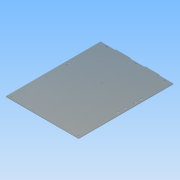
# Autodesk Inventor part: задняя  панель new
Saved by Autodesk Inventor 2017 (Build 210142000, 142)
## iProperties
Part Number: задняя  панель new
Material: Типовые
Document SubType Name: Modeling
Designer: Max
Mass: 792.41 g
Surface Area: 4047.62 cm^2
Volume: 792.41 cm^3
Density: 1 g/cm^3
Appearance: Поликарбонат — дымчатый
Author: Max
Autodesk Inventor part; units mm, degrees
ref_plane "YZ Plane" through (0, 0, 0) normal (1, 0, 0) x (0, 1, 0)
ref_plane "XZ Plane" through (0, 0, 0) normal (0, 1, 0) x (-1, 0, 0)
ref_plane "XY Plane" through (0, 0, 0) normal (0, 0, 1) x (1, 0, 0)
sketch "Эскиз1" plane through (0, 0, 0) normal (0, 0, 1) x (1, 0, 0)
  circle A0 centre (7.4641, 67.6713) radius 2
  circle A1 centre (7.4641, 364.6713) radius 2
  circle A2 centre (-351.5359, 364.6713) radius 2
  circle A3 centre (-351.5359, 67.6713) radius 2
  line L0 (-359.0359, 370.6713) -> (14.9641, 370.6713)
  line L1 (14.9641, 370.6713) -> (14.9641, 53.6713)
  line L2 (14.9641, 53.6713) -> (-359.0359, 53.6713)
  line L3 (-359.0359, 53.6713) -> (-359.0359, 370.6713)
  line L4 (-359.0359, 370.6713) -> (-367.0359, 370.6713)
  line L5 (-367.0359, 370.6713) -> (-367.0359, 53.6713)
  line L6 (-367.0359, 53.6713) -> (-359.0359, 53.6713)
  line L7 (-359.0359, 53.6713) -> (-359.0359, 370.6713)
  line L8 (14.9641, 370.6713) -> (22.9641, 370.6713)
  line L9 (22.9641, 370.6713) -> (22.9641, 53.6713)
  line L10 (22.9641, 53.6713) -> (14.9641, 53.6713)
  line L11 (14.9641, 53.6713) -> (14.9641, 370.6713)
  dimension "d4" = 374
  dimension "d6" = 317
  dimension "d7" = 14
  dimension "d40" = 7.5
  dimension "d41" = 297
  dimension "d42" = 7.5
  dimension "d43" = 7.5
  dimension "d44" = 297
  dimension "d45" = 6
  dimension "d46" = 359
  dimension "d47" = 14
  dimension "d48" = 359
  dimension "d66" = 8
  dimension "d67" = 8
  dimension "d68" = 390
  dimension "d92" = 4
  dimension "d93" = 4
  dimension "d94" = 4
  dimension "d95" = 4
  constraints: 24 end point, 6 parallel, 4 centre point, 3 horizontal, 3 perpendicular, 1 coincident, 1 point on line
  measures "d4" distance between parallel lines of L1 L3
  measures "d6" distance between parallel lines of L0 L2
  measures "d7" distance from line of A3.centre L2
  measures "d40" distance from line of L1 A0.centre
  measures "d41" distance of A0.centre A1.centre
  measures "d42" distance from line of L1 A1.centre
  measures "d43" distance from line of L3 A2.centre
  measures "d44" distance of A3.centre A2.centre
  measures "d45" distance from line of L0 A2.centre
  measures "d46" distance of A0.centre A3.centre
  measures "d47" distance from line of L2 A0.centre
  measures "d48" distance of A1.centre A2.centre
  measures "d66" distance between parallel lines of L9 L1
  measures "d67" distance between parallel lines of L7 L5
  measures "d68" distance between parallel lines of L5 L9
  measures "d92" diameter of A3
  measures "d93" diameter of A0
  measures "d94" diameter of A1
  measures "d95" diameter of A2
extrude "Выдавливание1" add sketch "Эскиз1" along normal blind 4
sketch "Эскиз3" plane through (0, 0, 4) normal (0, 0, 1) x (1, 0, 0)
  circle A0 centre (7.4641, 319.6713) radius 5
  circle A1 centre (7.4641, 282.6713) radius 5
  circle A2 centre (-351.5359, 254.6713) radius 2
  point P0 (0, 0)
  dimension "d96" = 10
  dimension "d97" = 10
  constraints: 3 centre point, 4 other
  measures "d96" diameter of A0
  measures "d97" diameter of A1
sketch "Эскиз4" plane through (0, 0, 4) normal (0, 0, 1) x (1, 0, 0)
  circle A0 centre (-171.5359, 372.6713) radius 1.5
  line L0 (-182.5359, 370.6713) -> (-179.0359, 378.6713)
  line L1 (-179.0359, 378.6713) -> (-164.0359, 378.6713)
  line L2 (-164.0359, 378.6713) -> (-160.5359, 370.6713)
  line L3 (22.9641, 370.6713) -> (-367.0359, 370.6713) projected
  line L4 (-171.5359, 372.6713) -> (-171.5359, 378.6713)
  circle A1 centre (-171.5359, 372.6713) radius 1.5
  point P0 (0, 0)
  point P1 (10.9641, 370.6713)
  point P2 (-363.0359, 370.6713)
  dimension "d49" = 8
  dimension "d50" = 22
  dimension "d51" = 15
  constraints: 8 end point, 2 centre point, 2 point on line, 1 coincident, 1 midpoint, 1 perpendicular, 1 symmetric about line, 2 other
  measures "d49" distance between parallel lines of L3 L1
  measures "d50" distance of L0.start L2.end
  measures "d51" distance of L0.end L1.end
sketch "Эскиз5" plane through (0, 0, 0) normal (0, 0, -1) x (-1, 0, 0)
  line L0 (-22.9641, 370.6713) -> (367.0359, 370.6713)
  line L1 (-22.9641, 370.6713) -> (367.0359, 370.6713)
  line L2 (367.0359, 370.6713) -> (367.0359, 561.6713)
  line L3 (367.0359, 561.6713) -> (-22.9641, 561.6713)
  line L4 (-22.9641, 561.6713) -> (-22.9641, 370.6713)
  line L5 (367.0359, 370.6713) -> (367.0359, 53.6713) projected
  line L6 (-22.9641, 53.6713) -> (-22.9641, 370.6713) projected
  point P0 (0, 0)
  point P1 (363.0359, 370.6713)
  dimension "d69" = 390
  dimension "d70" = 191
  constraints: 10 end point, 2 collinear, 2 parallel, 1 horizontal, 1 perpendicular
  measures "d69" distance between parallel lines of L2 L4
  measures "d70" distance between parallel lines of L0 L3
extrude "Выдавливание4" add sketch "Эскиз5" against normal blind 4
extrude "Выдавливание5" cut sketch "Эскиз3" against normal blind 4
extrude "Выдавливание6" cut sketch "Эскиз4" against normal blind 5 contours A0
sketch "Эскиз7" plane through (0, 0, 4) normal (0, 0, 1) x (1, 0, 0)
  circle A0 centre (-353.0359, 403.6713) radius 3.75 construction
  circle A1 centre (-351.0359, 376.6713) radius 3.75 construction
  circle A2 centre (8.9641, 403.6713) radius 3.75 construction
  circle A3 centre (6.9641, 376.6713) radius 3.75 construction
  circle A4 centre (8.9641, 403.6713) radius 5
  circle A5 centre (6.9641, 376.6713) radius 5
  circle A6 centre (-353.0359, 403.6713) radius 5
  circle A7 centre (-351.0359, 376.6713) radius 5
  point P0 (0, 0)
  dimension "d71" = 10
  dimension "d72" = 10
  dimension "d73" = 10
  dimension "d74" = 10
  constraints: 4 centre point, 4 coincident
  measures "d71" diameter of A4
  measures "d72" diameter of A5
  measures "d73" diameter of A6
  measures "d74" diameter of A7
extrude "Выдавливание8" cut sketch "Эскиз7" against normal blind 10
sketch "Эскиз8" plane through (0, 0, 4) normal (0, 0, 1) x (1, 0, 0)
  line L0 (-367.0359, 53.6713) -> (-367.0359, 561.6713) projected
  line L1 (-367.0359, 561.6713) -> (-289.0359, 561.6713)
  line L2 (-289.0359, 561.6713) -> (-289.0359, 565.6713)
  line L3 (-289.0359, 565.6713) -> (-367.0359, 565.6713)
  line L4 (-367.0359, 565.6713) -> (-367.0359, 561.6713)
  line L5 (-367.0359, 561.6713) -> (22.9641, 561.6713) projected
  line L6 (-288.7359, 565.6713) -> (-211.3359, 565.6713)
  line L7 (-211.3359, 565.6713) -> (-211.3359, 561.6713)
  line L8 (-211.3359, 561.6713) -> (-288.7359, 561.6713)
  line L9 (-288.7359, 561.6713) -> (-288.7359, 565.6713)
  line L10 (-211.0359, 565.6713) -> (-133.0359, 565.6713)
  line L11 (-133.0359, 565.6713) -> (-133.0359, 561.6713)
  line L12 (-133.0359, 561.6713) -> (-211.0359, 561.6713)
  line L13 (-211.0359, 561.6713) -> (-211.0359, 565.6713)
  line L14 (22.9641, 561.6713) -> (-367.0359, 561.6713) projected
  line L15 (-132.7359, 561.6713) -> (-55.3359, 561.6713)
  line L16 (-55.3359, 561.6713) -> (-55.3359, 565.6713)
  line L17 (-55.3359, 565.6713) -> (-132.7359, 565.6713)
  line L18 (-132.7359, 565.6713) -> (-132.7359, 561.6713)
  line L19 (22.9641, 561.6713) -> (-55.0359, 561.6713)
  line L20 (-55.0359, 561.6713) -> (-55.0359, 565.6713)
  line L21 (-55.0359, 565.6713) -> (22.9641, 565.6713)
  line L22 (22.9641, 565.6713) -> (22.9641, 561.6713)
  point P0 (0, 0)
  dimension "d77" = 78
  dimension "d78" = 4
  dimension "d79" = 4
  dimension "d80" = 0.3
  dimension "d81" = 0.3
  dimension "d82" = 77.4
  dimension "d83" = 78
  dimension "d84" = 0.3
  dimension "d85" = 4
  dimension "d86" = 77.4
  dimension "d87" = 4
  dimension "d88" = 0.3
  dimension "d89" = 78
  constraints: 40 end point, 10 parallel, 5 horizontal, 5 perpendicular, 3 point on line, 1 collinear
  measures "d77" distance between parallel lines of L4 L2
  measures "d78" distance between parallel lines of L1 L3
  measures "d79" distance between parallel lines of L1 L6
  measures "d80" distance between parallel lines of L2 L9
  measures "d81" distance between parallel lines of L13 L7
  measures "d82" distance between parallel lines of L7 L9
  measures "d83" distance between parallel lines of L11 L13
  measures "d84" distance between parallel lines of L11 L18
  measures "d85" distance between parallel lines of L5 L17
  measures "d86" distance between parallel lines of L18 L16
  measures "d87" distance between parallel lines of L19 L21
  measures "d88" distance between parallel lines of L16 L20
  measures "d89" distance between parallel lines of L22 L20
extrude "Выдавливание9" add sketch "Эскиз8" against normal blind 4 contours L18 L17 L16 L5 | L9 L6 L7 L5
sketch "Эскиз10" plane through (0, 0, 4) normal (0, 0, 1) x (1, 0, 0)
  line L0 (-329.3859, 556.6713) -> (-329.3859, 561.6713) projected
  line L1 (-330.6859, 556.6713) -> (-329.3859, 556.6713)
  line L2 (-330.6859, 554.2213) -> (-330.6859, 556.6713)
  line L3 (-329.3859, 554.2213) -> (-330.6859, 554.2213)
  line L4 (-326.3859, 553.1713) -> (-329.3859, 553.1713)
  line L5 (-329.3859, 553.1713) -> (-329.3859, 554.2213)
  line L6 (-326.3859, 554.2213) -> (-326.3859, 553.1713)
  line L7 (-325.0859, 554.2213) -> (-326.3859, 554.2213)
  line L8 (-325.0859, 556.6713) -> (-325.0859, 554.2213)
  line L9 (-326.3859, 556.6713) -> (-325.0859, 556.6713)
  line L10 (-326.3859, 561.6713) -> (-326.3859, 556.6713) projected
  line L11 (-173.5359, 556.6713) -> (-173.5359, 561.6713) projected
  line L12 (-170.5359, 561.6713) -> (-170.5359, 556.6713) projected
  line L13 (-174.8359, 556.6713) -> (-173.5359, 556.6713)
  line L14 (-174.8359, 554.2213) -> (-174.8359, 556.6713)
  line L15 (-173.5359, 554.2213) -> (-174.8359, 554.2213)
  line L16 (-173.5359, 553.1713) -> (-173.5359, 554.2213)
  line L17 (-170.5359, 553.1713) -> (-173.5359, 553.1713)
  circle A0 centre (-353.0359, 403.6713) radius 5 projected
  circle A1 centre (8.9641, 403.6713) radius 5 projected
  circle A2 centre (6.9641, 376.6713) radius 5 projected
  circle A3 centre (-351.0359, 376.6713) radius 5 projected
  circle A4 centre (-171.5359, 372.6713) radius 1.5 projected
  circle A5 centre (7.4641, 319.6713) radius 5 projected
  circle A6 centre (-351.5359, 254.6713) radius 2 projected
  circle A7 centre (7.4641, 282.6713) radius 5 projected
  circle A8 centre (-351.5359, 67.6713) radius 2 projected
  circle A9 centre (-351.5359, 364.6713) radius 2 projected
  circle A10 centre (7.4641, 364.6713) radius 2 projected
  circle A11 centre (7.4641, 67.6713) radius 2 projected
  line L18 (-367.0359, 561.6713) -> (-367.0359, 53.6713) projected
  line L19 (-367.0359, 53.6713) -> (22.9641, 53.6713) projected
  line L20 (22.9641, 53.6713) -> (22.9641, 561.6713) projected
  line L21 (22.9641, 561.6713) -> (-55.3359, 561.6713) projected
  line L22 (-55.3359, 561.6713) -> (-55.3359, 565.6713) projected
  line L23 (-55.3359, 565.6713) -> (-132.7359, 565.6713) projected
  line L24 (-132.7359, 565.6713) -> (-132.7359, 561.6713) projected
  line L25 (-132.7359, 561.6713) -> (-211.3359, 561.6713) projected
  line L26 (-211.3359, 561.6713) -> (-211.3359, 565.6713) projected
  line L27 (-211.3359, 565.6713) -> (-288.7359, 565.6713) projected
  line L28 (-288.7359, 565.6713) -> (-288.7359, 561.6713) projected
  line L29 (-288.7359, 561.6713) -> (-367.0359, 561.6713) projected
  line L30 (-169.2359, 554.2213) -> (-170.5359, 554.2213)
  line L31 (-169.2359, 556.6713) -> (-169.2359, 554.2213)
  line L32 (-170.5359, 556.6713) -> (-169.2359, 556.6713)
  line L33 (-170.5359, 554.2213) -> (-170.5359, 553.1713)
  line L34 (-17.6859, 556.6713) -> (-17.6859, 561.6713) projected
  line L35 (-14.6859, 561.6713) -> (-14.6859, 556.6713) projected
  line L36 (-14.6859, 556.6713) -> (-13.3859, 556.6713)
  line L37 (-13.3859, 556.6713) -> (-13.3859, 554.2213)
  line L38 (-13.3859, 554.2213) -> (-14.6859, 554.2213)
  line L39 (-14.6859, 554.2213) -> (-14.6859, 553.1713)
  line L40 (-14.6859, 553.1713) -> (-17.6859, 553.1713)
  line L41 (-17.6859, 553.1713) -> (-17.6859, 554.2213)
  line L42 (-17.6859, 554.2213) -> (-18.9859, 554.2213)
  line L43 (-18.9859, 554.2213) -> (-18.9859, 556.6713)
  line L44 (-18.9859, 556.6713) -> (-17.6859, 556.6713)
  line L45 (-17.6859, 561.6713) -> (-14.6859, 561.6713)
  line L46 (-55.3359, 561.6713) -> (22.9641, 561.6713) projected
  line L47 (-173.5359, 561.6713) -> (-170.5359, 561.6713)
  line L48 (-329.3859, 561.6713) -> (-326.3859, 561.6713)
  line L49 (-288.7359, 561.6713) -> (-367.0359, 561.6713) projected
  point P0 (0, 0)
  dimension "d100" = 1.3
  dimension "d101" = 1.3
  dimension "d102" = 1.3
  dimension "d103" = 1.3
  dimension "d104" = 1.3
  dimension "d105" = 1.3
  dimension "d106" = 5
  dimension "d107" = 1.3
  dimension "d108" = 2.45
  dimension "d109" = 8.5
  dimension "d110" = 8.5
  dimension "d111" = 8.5
  constraints: 60 end point, 19 collinear
  measures "d100" distance between parallel lines of L0 L2
  measures "d101" distance between parallel lines of L8 L10
  measures "d102" distance between parallel lines of L11 L14
  measures "d103" distance between parallel lines of L31 L12
  measures "d104" distance between parallel lines of L34 L43
  measures "d105" distance between parallel lines of L35 L37
  measures "d106" distance between parallel lines of L21 L44
  measures "d107" distance of L43.end L34.start
  measures "d108" distance between parallel lines of L44 L42
  measures "d109" distance between parallel lines of L25 L17
  measures "d110" distance between parallel lines of L21 L40
  measures "d111" distance between parallel lines of L29 L4
extrude "Выдавливание10" cut sketch "Эскиз10" against normal blind 10 contours L0 L29 L10 L9 L8 L7 L6 L4 L5 L3 L2 L1 | L35 L36 L37 L38 L39 L40 L41 L42 L43 L44 L34 L21 | L25 L12 L32 L31 L30 L33 L17 L16 L15 L14 L13 L11
